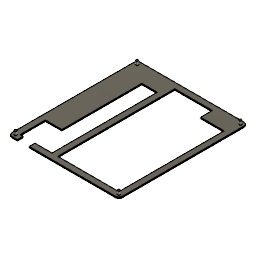
EasySplit-Right-Assembled (Autodesk Fusion 360 archive; units mm, degrees)
design "EasySplit-Right-Top"
part number: 2026-04-16-19-10-06-869
Autodesk Fusion 360 part; units mm, degrees
note: some values were not read from the file. Chosen so that the rebuilt part matches the saved one: a side.
(part 1 of 2)
sketch "Sketch1" plane through (0, 0, 0) normal (0, 0, 1) x (1, 0, 0)
  line L0 (167.6875, -193.6438) -> (-20, -193.6438)
  line L1 (-10, 15) -> (157.6875, 15)
  line L2 (-20, -193.6438) -> (-20, 25)
  line L3 (167.6875, 25) -> (167.6875, -193.6438)
  line L4 (-10, -183.6438) -> (-10, 15)
  line L5 (157.6875, 15) -> (157.6875, -183.6438)
  line L6 (157.6875, -183.6438) -> (-10, -183.6438)
  line L7 (-20, 25) -> (167.6875, 25)
  line L8 (15, -183.6438) -> (-5, -183.6438)
  line L9 (-5, -183.6438) -> (-5, -193.6438)
  line L10 (-5, -193.6438) -> (15, -193.6438)
  line L11 (15, -193.6438) -> (15, -183.6438)
  line L12 (-10, 15) -> (18, 15)
  line L13 (18, 15) -> (18, -141)
  line L14 (18, -141) -> (-10, -141)
  line L15 (-10, -141) -> (-10, 15)
  line L16 (44, 15) -> (54, 15)
  line L17 (54, 15) -> (54, -185)
  line L18 (54, -185) -> (44, -185)
  line L19 (44, -185) -> (44, 15)
  line L20 (157.6875, -183.6438) -> (121.6875, -183.6438)
  line L21 (121.6875, -183.6438) -> (121.6875, -148.1438)
  line L22 (121.6875, -148.1438) -> (157.6875, -148.1438)
  line L23 (157.6875, -148.1438) -> (157.6875, -183.6438)
  line L24 (18, -141) -> (44, -141)
  line L25 (14, -141) -> (18, -141)
  line L26 (18, 15) -> (44, 15)
  line L27 (44, 15) -> (44, -5)
  line L28 (44, -5) -> (18, -5)
  line L29 (18, -5) -> (18, 15)
  line L30 (157.6875, 15) -> (117.6875, 15)
  line L31 (117.6875, 15) -> (117.6875, -5)
  line L32 (117.6875, -5) -> (157.6875, -5)
  line L33 (157.6875, -5) -> (157.6875, 15)
  dimension "d3" = 167.6875
  dimension "d4" = 198.6438
  dimension "d5" = 187.6875
  dimension "d6" = 218.6438
  dimension "d7" = 10
  dimension "d8" = 10
  dimension "d19" = 20
  dimension "d20" = 15
  dimension "d21" = 28
  dimension "d22" = 156
  dimension "d23" = 10
  dimension "d24" = 200
  dimension "d25" = 26
  dimension "d26" = 36
  dimension "d27" = 35.5
  dimension "d29" = 10
  dimension "d30" = 20
  dimension "d31" = 40
  dimension "d32" = 20
  constraint horizontal L1
  constraint vertical L5
  constraint horizontal L6
  constraint vertical L4
  constraint horizontal L7
  constraint vertical L3
  constraint horizontal L0
  constraint vertical L2
  constraint horizontal L8
  constraint vertical L9
  constraint horizontal L10
  constraint vertical L11
  constraint coincident L6 L8.start
  constraint horizontal L12
  constraint vertical L13
  constraint horizontal L14
  constraint vertical L15
  constraint horizontal L16
  constraint vertical L17
  constraint horizontal L18
  constraint vertical L19
  constraint coincident L1 L16.start
  constraint horizontal L20
  constraint vertical L21
  constraint horizontal L22
  constraint vertical L23
  constraint horizontal L24
  constraint horizontal L25
  constraint coincident L14 L25.start
  constraint horizontal L26
  constraint vertical L27
  constraint horizontal L28
  constraint vertical L29
  constraint horizontal L30
  constraint vertical L31
  constraint horizontal L32
  constraint vertical L33
  measures "d3" distance of L1.start L1.end
  measures "d4" distance of L1.start L4.start
  measures "d5" distance of L2.end L3.start
  measures "d6" distance of L2.end L0.end
  measures "d7" distance of L1 L7
  measures "d8" distance of L2 L4
  measures "d19" distance of L8.start L8.end
  measures "d20" distance of L2 L9
  measures "d21" distance of L1.start L12.end
  measures "d22" distance of L1.start L14.end
  measures "d23" distance of L16.start L16.end
  measures "d24" distance of L16.start L18.end
  measures "d25" distance of L13 L19
  measures "d26" distance of L5.end L20.end
  measures "d27" distance of L5.end L22.end
  measures "d29" distance of L8.start L10.end
  measures "d30" distance of L12.end L28.end
  measures "d31" distance of L1.end L30.end
  measures "d32" distance of L1.end L32.end
extrude "Extrude1" add sketch "Sketch1" along normal blind 2 contours L0 L1 L2 L3 L4 L5 L6 L7 L9 L11 L12 L15 L16 L17 L18 L19 L20 L23 L26 L30 L33 | L1 L6 L16 L17 L19 L27 | L6 L17 L18 L19 | L1 L4 L12 L13 L14 L15 L25 L29 | L1 L13 L19 L26 L27 L28 L29 | L1 L5 L30 L31 L32 L33
fillet "Fillet1" radius 6 1 edges at (167.6875, -193.6438, 1)
fillet "Fillet2" radius 6 1 edges at (167.6875, 25, 1)
fillet "Fillet3" radius 6 1 edges at (-20, 25, 1)
fillet "Fillet4" radius 6 1 edges at (-20, -193.6438, 1)
move_face "MoveFace1" to x (-1, 0, 0) y (0, 1, 0) z (0, 0, -1) at (108, 0, 4) 1 faces at (-4, -42.3333, 2)
sketch "Sketch2" plane through (0, 0, 2) normal (0, 0, 1) x (-1, 0, 0)
  arc A0 (20, 187.6438) -> (14, 193.6438) centre (14, 187.6438) ccw
  line L0 (14, 193.6438) -> (5, 193.6438)
  line L1 (5, 193.6438) -> (5, 183.6438)
  line L2 (5, 183.6438) -> (10, 183.6438)
  line L3 (10, 183.6438) -> (10, 141)
  line L4 (10, 141) -> (-18, 141)
  line L5 (-18, 141) -> (-18, 5)
  line L6 (-18, 5) -> (-44, 5)
  line L7 (-44, 5) -> (-44, 183.6438)
  line L8 (-44, 183.6438) -> (-15, 183.6438)
  line L9 (-15, 183.6438) -> (-15, 193.6438)
  line L10 (-15, 193.6438) -> (-161.6875, 193.6438)
  arc A1 (-161.6875, 193.6438) -> (-167.6875, 187.6438) centre (-161.6875, 187.6438) ccw
  line L11 (-167.6875, 187.6438) -> (-167.6875, -19)
  arc A2 (-167.6875, -19) -> (-161.6875, -25) centre (-161.6875, -19) ccw
  line L12 (-161.6875, -25) -> (14, -25)
  arc A3 (14, -25) -> (20, -19) centre (14, -19) ccw
  line L13 (20, -19) -> (20, 187.6438)
  line L14 (-54, 183.6438) -> (-54, -15)
  line L15 (-54, -15) -> (-117.6875, -15)
  line L16 (-117.6875, -15) -> (-117.6875, 5)
  line L17 (-117.6875, 5) -> (-157.6875, 5)
  line L18 (-157.6875, 5) -> (-157.6875, 183.6438)
  line L19 (-157.6875, 183.6438) -> (-54, 183.6438)
  circle A4 centre (14, -19) radius 2.1
  circle A5 centre (-161.6875, -19) radius 2.1
  circle A6 centre (-161.6875, 187.6438) radius 2.1
  circle A7 centre (14, 187.6438) radius 2.1
  dimension "d33" = 4.2
  dimension "d34" = 4.2
  dimension "d35" = 4.2
  dimension "d36" = 4.2
  dimension "d37" = 6
  dimension "d38" = 6
  dimension "d39" = 6
  dimension "d40" = 6
  dimension "d41" = 6
  dimension "d42" = 6
  dimension "d43" = 6
  dimension "d44" = 6
  measures "d33" diameter of A4
  measures "d34" diameter of A5
  measures "d35" diameter of A6
  measures "d36" diameter of A7
  measures "d37" distance of L0 A0.centre
  measures "d38" distance of L13 A0.centre
  measures "d39" distance of L13 A3.centre
  measures "d40" distance of L12 A3.centre
  measures "d41" distance of L11 A2.centre
  measures "d42" distance of L12 A2.centre
  measures "d43" distance of L10 A1.centre
  measures "d44" distance of L11 A1.centre
extrude "Extrude2" add sketch "Sketch2" along normal blind 6 contours A4 | A5 | A6 | A7

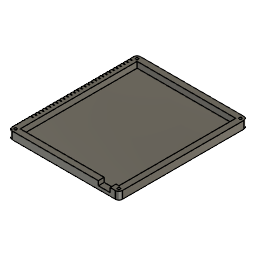
design "EasySplit-Right"
part number: 2026-04-16-18-11-24-138
Autodesk Fusion 360 part; units mm, degrees
sketch "Sketch1" plane through (0, 0, 0) normal (0, 0, 1) x (1, 0, 0)
  line L0 (-10, 15) -> (157.6875, 15)
  line L1 (157.6875, 15) -> (157.6875, -183.6438)
  line L2 (157.6875, -183.6438) -> (-10, -183.6438)
  line L3 (-10, -183.6438) -> (-10, 15)
  line L4 (-20, 25) -> (167.6875, 25)
  line L5 (167.6875, 25) -> (167.6875, -193.6438)
  line L6 (167.6875, -193.6438) -> (-20, -193.6438)
  line L7 (-20, -193.6438) -> (-20, 25)
  dimension "d1" = 167.6875
  dimension "d2" = 198.6438
  dimension "d3" = 187.6875
  dimension "d4" = 218.6438
  dimension "d5" = 10
  dimension "d6" = 10
  constraint horizontal L0
  constraint vertical L1
  constraint horizontal L2
  constraint vertical L3
  constraint horizontal L4
  constraint vertical L5
  constraint horizontal L6
  constraint vertical L7
  measures "d1" distance of L0.start L0.end
  measures "d2" distance of L0.start L2.end
  measures "d3" distance of L4.start L4.end
  measures "d4" distance of L4.start L6.end
  measures "d5" distance of L0 L4
  measures "d6" distance of L3 L7
extrude "Extrude1" add sketch "Sketch1" along normal blind 3 contours L0 L1 L2 L3
extrude "Extrude2" add sketch "Sketch1" along normal blind 13
sketch "Sketch2" plane through (0, 0, 13) normal (0, 0, 1) x (-1, 0, 0)
  line L0 (-157.6875, 183.6438) -> (10, 183.6438)
  line L1 (10, 183.6438) -> (10, -15)
  line L2 (10, -15) -> (-157.6875, -15)
  line L3 (-157.6875, -15) -> (-157.6875, 183.6438)
  line L4 (20, 193.6438) -> (-167.6875, 193.6438)
  line L5 (-167.6875, 193.6438) -> (-167.6875, -25)
  line L6 (-167.6875, -25) -> (20, -25)
  line L7 (20, -25) -> (20, 193.6438)
  line L8 (20, -25) -> (-167.6875, -25)
  line L9 (-132.6875, 183.6438) -> (-152.6875, 183.6438)
  line L10 (-152.6875, 183.6438) -> (-152.6875, 193.6438)
  line L11 (-152.6875, 193.6438) -> (-132.6875, 193.6438)
  line L12 (-132.6875, 193.6438) -> (-132.6875, 183.6438)
  line L13 (20, 193.6438) -> (20, -25)
  dimension "d15" = 20
  dimension "d21" = 15
  constraint horizontal L9
  constraint vertical L10
  constraint horizontal L11
  constraint vertical L12
  constraint coincident L0 L9.start
  measures "d15" distance of L9.start L9.end
  measures "d21" distance of L5 L10
extrude "Extrude4" cut sketch "Sketch2" against normal blind 7.5 contours L0 L4 L9 L10 L11 L12
fillet "Fillet1" radius 6 4 edges at (-20, -193.6438, 6.5) (167.6875, -193.6438, 6.5) (167.6875, 25, 6.5) (-20, 25, 6.5)
sketch "Sketch3" plane through (-20, 0, 0) normal (-1, 0, 0) x (0, -1, 0)
  line L0 (-19, 13) -> (-19, 0)
  line L1 (-19, 0) -> (187.6438, 0)
  line L2 (187.6438, 0) -> (187.6438, 13)
  line L3 (187.6438, 13) -> (-19, 13)
  line L4 (149, 0) -> (156.5042, 12.9976)
  line L5 (23, 0) -> (30.5042, 12.9976)
  line L6 (167, 0) -> (174.5042, 12.9976)
  line L7 (179, 0) -> (186.5042, 12.9976)
  line L8 (77, 0) -> (84.5042, 12.9976)
  line L9 (113, 0) -> (120.5042, 12.9976)
  line L10 (71, 0) -> (78.5042, 12.9976)
  line L11 (41, 0) -> (48.5042, 12.9976)
  line L12 (173, 0) -> (180.5042, 12.9976)
  line L13 (143, 0) -> (150.5042, 12.9976)
  line L14 (65, 0) -> (72.5042, 12.9976)
  line L15 (131, 0) -> (138.5042, 12.9976)
  line L16 (29, 0) -> (36.5042, 12.9976)
  line L17 (101, 0) -> (108.5042, 12.9976)
  line L18 (107, 0) -> (114.5042, 12.9976)
  line L19 (35, 0) -> (42.5042, 12.9976)
  line L20 (47, 0) -> (54.5042, 12.9976)
  line L21 (53, 0) -> (60.5042, 12.9976)
  line L22 (59, 0) -> (66.5042, 12.9976)
  line L23 (137, 0) -> (144.5042, 12.9976)
  line L24 (155, 0) -> (162.5042, 12.9976)
  line L25 (89, 0) -> (96.5042, 12.9976)
  line L26 (161, 0) -> (168.5042, 12.9976)
  line L27 (83, 0) -> (90.5042, 12.9976)
  line L28 (125, 0) -> (132.5042, 12.9976)
  line L29 (95, 0) -> (102.5042, 12.9976)
  line L30 (119, 0) -> (126.5042, 12.9976)
  line L31 (17, 0) -> (24.5042, 12.9976)
  line L32 (11, 0) -> (18.5042, 12.9976)
  line L33 (5, 0) -> (12.5042, 12.9976)
  line L34 (-1, 0) -> (6.5042, 12.9976)
  line L35 (-7, 0) -> (0.5042, 12.9976)
  line L36 (-13, 0) -> (-5.4958, 12.9976)
  line L37 (-19, 0) -> (-11.4958, 12.9976)
  line L38 (185, 0) -> (192.5042, 12.9976)
  spline S0 degree 2 poles (-161.6453, 5.852) (-161.6453, 5.4239) (-161.4102, 5.1797) knots 0 0 0 1 1 1
  spline S1 degree 2 poles (-158.3964, 3.5539) (-158.3964, 3.399) (-158.3281, 3.2729) knots 0 0 0 1 1 1
  spline S2 degree 2 poles (-160.7602, 4.9354) (-160.3925, 4.9354) (-160.1219, 5.156) knots 0 0 0 1 1 1
  spline S3 degree 2 poles (-171.3603, 5.7785) (-171.3603, 6.6006) (-170.8621, 7.2256) knots 0 0 0 1 1 1
  spline S4 degree 2 poles (-158.8179, 7.9781) (-158.9269, 8.0871) (-158.9926, 8.3839) knots 0 0 0 1 1 1
  spline S5 degree 2 poles (-171.1933, 5.118) (-171.3603, 5.3661) (-171.3603, 5.7785) knots 0 0 0 1 1 1
  line L39 (-149.6321, 8.0608) -> (-148.2454, 8.0608)
  spline S6 degree 2 poles (-150.1259, 8.2426) (-150.0051, 8.6482) (-149.837, 8.7997) knots 0 0 0 1 1 1
  line L40 (-150.2782, 7.722) -> (-150.7221, 7.722)
  spline S7 degree 2 poles (-152.3531, 8.4044) (-152.1771, 8.4123) (-151.8475, 8.5819) knots 0 0 0 1 1 1
  line L41 (-152.3898, 8.4071) -> (-152.3531, 8.4044)
  spline S8 degree 2 poles (-156.29, 5.4712) (-156.8022, 4.9354) (-157.5061, 4.9354) knots 0 0 0 1 1 1
  spline S9 degree 2 poles (-158.4095, 8.2552) (-157.9237, 8.2552) (-157.4745, 8.4338) knots 0 0 0 1 1 1
  spline S10 degree 2 poles (-157.5061, 4.9354) (-157.8869, 4.9354) (-158.139, 5.0983) knots 0 0 0 1 1 1
  line L42 (-157.4745, 8.4338) -> (-157.6768, 7.42)
  line L43 (-150.575, 8.0608) -> (-150.1784, 8.0608)
  spline S11 degree 2 poles (-154.575, 6.3773) (-154.6564, 5.9518) (-154.6564, 5.7916) knots 0 0 0 1 1 1
  spline S12 degree 2 poles (-152.8468, 7.3523) (-152.5054, 7.431) (-152.4187, 7.431) knots 0 0 0 1 1 1
  spline S13 degree 2 poles (-164.0195, 7.1258) (-164.5842, 6.3694) (-165.4929, 5.8599) knots 0 0 0 1 1 1
  spline S14 degree 2 poles (-165.1147, 3.9348) (-164.3452, 3.9348) (-163.6439, 4.9512) knots 0 0 0 1 1 1
  spline S15 degree 2 poles (-164.248, 3.8783) (-164.7917, 3.4436) (-165.183, 3.4436) knots 0 0 0 1 1 1
  line L44 (-165.8632, 6.506) -> (-165.6295, 6.0805)
  spline S16 degree 2 poles (-166.6459, 7.1626) (-166.6459, 7.6616) (-166.0655, 7.9663) knots 0 0 0 1 1 1
  spline S17 degree 2 poles (-166.9795, 4.6176) (-167.1659, 4.7542) (-167.1659, 4.9459) knots 0 0 0 1 1 1
  spline S18 degree 2 poles (-165.4036, 5.4791) (-165.4036, 5.0772) (-165.7398, 4.7791) knots 0 0 0 1 1 1
  spline S19 degree 2 poles (-166.7116, 4.9801) (-166.7116, 4.7647) (-166.399, 4.7647) knots 0 0 0 1 1 1
  spline S20 degree 2 poles (-166.9099, 5.3609) (-166.6538, 5.571) (-166.0523, 5.8599) knots 0 0 0 1 1 1
  spline S21 degree 2 poles (-166.399, 4.7647) (-166.1679, 4.7647) (-166.0235, 4.921) knots 0 0 0 1 1 1
  line L45 (-166.0523, 5.8599) -> (-166.2625, 6.1987)
  spline S22 degree 2 poles (-165.9394, 5.6235) (-166.7116, 5.2086) (-166.7116, 4.9801) knots 0 0 0 1 1 1
  line L46 (-166.5277, 7.2309) -> (-166.3229, 7.0891)
  spline S23 degree 2 poles (-165.4929, 5.8599) (-165.4036, 5.6603) (-165.4036, 5.4791) knots 0 0 0 1 1 1
  spline S24 degree 2 poles (-167.1659, 4.9459) (-167.1659, 5.1508) (-166.9099, 5.3609) knots 0 0 0 1 1 1
  spline S25 degree 2 poles (-166.2625, 6.1987) (-166.6459, 6.8159) (-166.6459, 7.1626) knots 0 0 0 1 1 1
  spline S26 degree 2 poles (-165.7398, 4.7791) (-166.076, 4.4811) (-166.5277, 4.4811) knots 0 0 0 1 1 1
  spline S27 degree 2 poles (-166.0655, 7.9663) (-165.7083, 7.8297) (-165.7083, 7.6222) knots 0 0 0 1 1 1
  spline S28 degree 2 poles (-160.8153, 7.9584) (-160.8153, 7.764) (-160.7431, 7.6616) knots 0 0 0 1 1 1
  line L47 (-158.139, 5.0983) -> (-158.3307, 4.1265)
  spline S29 degree 2 poles (-159.8514, 5.6734) (-159.8514, 5.9912) (-160.4476, 6.548) knots 0 0 0 1 1 1
  spline S30 degree 2 poles (-161.2907, 7.764) (-161.2907, 8.2683) (-160.8967, 8.594) knots 0 0 0 1 1 1
  spline S31 degree 2 poles (-160.965, 4.6281) (-161.4141, 4.6281) (-161.707, 4.8382) knots 0 0 0 1 1 1
  line L48 (-160.4476, 6.548) -> (-160.7365, 6.8159)
  spline S32 degree 2 poles (-160.7365, 6.8159) (-161.2907, 7.3307) (-161.2907, 7.764) knots 0 0 0 1 1 1
  spline S33 degree 2 poles (-163.6807, 6.7608) (-163.4049, 6.007) (-163.2684, 5.395) knots 0 0 0 1 1 1
  spline S34 degree 2 poles (-158.9926, 8.3839) (-158.8009, 8.2552) (-158.4095, 8.2552) knots 0 0 0 1 1 1
  line L49 (-164.2296, 7.2545) -> (-164.0195, 7.1258)
  spline S35 degree 2 poles (-159.313, 8.2053) (-159.5415, 8.6465) (-160.0563, 8.6465) knots 0 0 0 1 1 1
  spline S36 degree 2 poles (-158.4804, 7.8691) (-158.7089, 7.8691) (-158.8179, 7.9781) knots 0 0 0 1 1 1
  spline S37 degree 2 poles (-158.097, 7.9164) (-158.3255, 7.8691) (-158.4804, 7.8691) knots 0 0 0 1 1 1
  spline S38 degree 2 poles (-160.1219, 5.156) (-159.8514, 5.3767) (-159.8514, 5.6734) knots 0 0 0 1 1 1
  spline S39 degree 2 poles (-164.2664, 7.5592) (-164.0904, 7.5592) (-163.9736, 7.4003) knots 0 0 0 1 1 1
  spline S40 degree 2 poles (-161.9998, 5.3688) (-161.9998, 5.5868) (-161.6453, 5.852) knots 0 0 0 1 1 1
  spline S41 degree 2 poles (-158.3281, 3.2729) (-158.5934, 3.1862) (-158.7326, 3.1862) knots 0 0 0 1 1 1
  spline S42 degree 2 poles (-161.707, 4.8382) (-161.9998, 5.0484) (-161.9998, 5.3688) knots 0 0 0 1 1 1
  spline S43 degree 2 poles (-158.9506, 3.4331) (-158.9506, 3.6248) (-158.8639, 4.0608) knots 0 0 0 1 1 1
  spline S44 degree 2 poles (-160.8967, 8.594) (-160.5028, 8.9197) (-159.8934, 8.9197) knots 0 0 0 1 1 1
  spline S45 degree 2 poles (-159.8934, 8.9197) (-159.5704, 8.9197) (-159.3708, 8.8212) knots 0 0 0 1 1 1
  spline S46 degree 2 poles (-159.8541, 4.9945) (-160.2953, 4.6281) (-160.965, 4.6281) knots 0 0 0 1 1 1
  spline S47 degree 2 poles (-173.6059, 4.8382) (-174.4647, 4.8382) (-174.4647, 5.4082) knots 0 0 0 1 1 1
  spline S48 degree 2 poles (-167.4338, 5.6432) (-168.0589, 5.0641) (-168.508, 5.0641) knots 0 0 0 1 1 1
  line L50 (-173.5887, 7.2046) -> (-173.0456, 7.2046)
  line L51 (-173.3275, 8.4994) -> (-173.5887, 7.2046)
  spline S49 degree 2 poles (-167.4955, 6.0241) (-167.0031, 6.4981) (-166.5277, 7.2309) knots 0 0 0 1 1 1
  line L52 (-172.4803, 8.4994) -> (-173.3275, 8.4994)
  spline S50 degree 2 poles (-173.1935, 5.2585) (-172.5212, 5.2585) (-172.009, 5.4975) knots 0 0 0 1 1 1
  spline S51 degree 2 poles (-172.9755, 4.8973) (-173.3852, 4.8382) (-173.6059, 4.8382) knots 0 0 0 1 1 1
  line L53 (-174.2257, 7.2046) -> (-174.139, 7.2046)
  spline S52 degree 2 poles (-173.8711, 5.6078) (-173.8711, 5.2585) (-173.1935, 5.2585) knots 0 0 0 1 1 1
  spline S53 degree 2 poles (-172.4003, 5.0116) (-172.5658, 4.9564) (-172.9755, 4.8973) knots 0 0 0 1 1 1
  spline S54 degree 2 poles (-174.4988, 8.7306) (-174.3202, 8.8225) (-173.3984, 8.8225) knots 0 0 0 1 1 1
  line L54 (-173.8816, 8.4994) -> (-173.9578, 8.4994)
  line L55 (-174.2047, 6.879) -> (-174.2441, 6.879)
  spline S55 degree 2 poles (-174.5212, 7.1258) (-174.4279, 7.2046) (-174.2257, 7.2046) knots 0 0 0 1 1 1
  spline S56 degree 2 poles (-174.4647, 5.4082) (-174.4647, 5.5605) (-174.3806, 5.9939) knots 0 0 0 1 1 1
  spline S57 degree 2 poles (-170.4826, 5.3714) (-170.1065, 5.3714) (-169.044, 7.0208) knots 0 0 0 1 1 1
  spline S58 degree 2 poles (-170.5404, 7.0457) (-170.8298, 6.5638) (-170.8298, 5.9019) knots 0 0 0 1 1 1
  spline S59 degree 2 poles (-159.4128, 5.9177) (-159.4128, 5.3609) (-159.8541, 4.9945) knots 0 0 0 1 1 1
  spline S60 degree 2 poles (-160.7431, 7.6616) (-160.6709, 7.5592) (-160.2953, 7.2151) knots 0 0 0 1 1 1
  spline S61 degree 2 poles (-163.9736, 7.4003) (-163.8567, 7.2414) (-163.6807, 6.7608) knots 0 0 0 1 1 1
  spline S62 degree 2 poles (-161.4102, 5.1797) (-161.1751, 4.9354) (-160.7602, 4.9354) knots 0 0 0 1 1 1
  spline S63 degree 2 poles (-164.0445, 6.3445) (-164.3321, 7.0339) (-164.6656, 7.3964) knots 0 0 0 1 1 1
  spline S64 degree 2 poles (-160.596, 8.4482) (-160.8153, 8.2499) (-160.8153, 7.9584) knots 0 0 0 1 1 1
  spline S65 degree 2 poles (-161.8475, 7.5434) (-161.8475, 7.2913) (-162.2611, 6.506) knots 0 0 0 1 1 1
  spline S66 degree 2 poles (-159.3708, 8.8212) (-159.1712, 8.7227) (-159.1712, 8.5651) knots 0 0 0 1 1 1
  spline S67 degree 2 poles (-163.6439, 4.9512) (-163.7569, 5.6551) (-164.0445, 6.3445) knots 0 0 0 1 1 1
  spline S68 degree 2 poles (-164.8731, 6.594) (-164.6183, 6.808) (-164.2296, 7.2545) knots 0 0 0 1 1 1
  spline S69 degree 2 poles (-162.2611, 6.506) (-162.6748, 5.7207) (-163.1528, 5.0667) knots 0 0 0 1 1 1
  line L56 (-158.8639, 4.0608) -> (-158.097, 7.9164)
  spline S70 degree 2 poles (-169.7092, 7.8507) (-169.3122, 7.8507) (-168.8495, 7.6038) knots 0 0 0 1 1 1
  spline S71 degree 2 poles (-170.8621, 7.2256) (-170.3639, 7.8507) (-169.7092, 7.8507) knots 0 0 0 1 1 1
  spline S72 degree 2 poles (-170.8298, 5.9019) (-170.8298, 5.3714) (-170.4826, 5.3714) knots 0 0 0 1 1 1
  spline S73 degree 2 poles (-168.1902, 7.8455) (-168.3399, 7.617) (-168.4187, 7.2204) knots 0 0 0 1 1 1
  spline S74 degree 2 poles (-169.044, 7.0208) (-169.0308, 7.0418) (-168.9361, 7.1679) knots 0 0 0 1 1 1
  spline S75 degree 2 poles (-169.8891, 5.357) (-170.3822, 4.8698) (-170.7476, 4.8698) knots 0 0 0 1 1 1
  spline S76 degree 2 poles (-170.7476, 4.8698) (-171.0264, 4.8698) (-171.1933, 5.118) knots 0 0 0 1 1 1
  spline S77 degree 2 poles (-168.2927, 7.8481) (-168.2611, 7.8481) (-168.1902, 7.8455) knots 0 0 0 1 1 1
  spline S78 degree 2 poles (-168.9361, 7.1679) (-169.4885, 7.5277) (-169.854, 7.5277) knots 0 0 0 1 1 1
  spline S79 degree 2 poles (-168.8495, 7.6038) (-168.7812, 7.8481) (-168.2927, 7.8481) knots 0 0 0 1 1 1
  line L57 (-168.4187, 7.2204) -> (-168.4634, 6.9971)
  spline S80 degree 2 poles (-169.0753, 6.0096) (-169.0753, 6.2066) (-169.0596, 6.5401) knots 0 0 0 1 1 1
  spline S81 degree 2 poles (-168.2716, 5.55) (-167.988, 5.55) (-167.4955, 6.0241) knots 0 0 0 1 1 1
  spline S82 degree 2 poles (-168.508, 5.0641) (-169.0753, 5.0641) (-169.0753, 6.0096) knots 0 0 0 1 1 1
  spline S83 degree 2 poles (-168.4634, 6.9971) (-168.5395, 6.6242) (-168.5395, 6.1252) knots 0 0 0 1 1 1
  spline S84 degree 2 poles (-169.854, 7.5277) (-170.2511, 7.5277) (-170.5404, 7.0457) knots 0 0 0 1 1 1
  spline S85 degree 2 poles (-168.5395, 6.1252) (-168.5395, 5.55) (-168.2716, 5.55) knots 0 0 0 1 1 1
  spline S86 degree 2 poles (-169.0596, 6.5401) (-169.3961, 5.8442) (-169.8891, 5.357) knots 0 0 0 1 1 1
  spline S87 degree 2 poles (-165.6295, 6.0805) (-165.1279, 6.3799) (-164.8731, 6.594) knots 0 0 0 1 1 1
  line L58 (-173.6521, 6.879) -> (-173.7867, 6.204)
  spline S88 degree 2 poles (-147.6886, 8.1557) (-147.7542, 7.8866) (-147.8632, 7.8043) knots 0 0 0 1 1 1
  spline S89 degree 2 poles (-172.6157, 8.8225) (-171.8751, 8.8225) (-171.4128, 8.9696) knots 0 0 0 1 1 1
  spline S90 degree 2 poles (-152.4187, 7.431) (-152.2244, 7.431) (-152.2244, 7.1581) knots 0 0 0 1 1 1
  spline S91 degree 2 poles (-172.4553, 6.9472) (-172.5944, 6.879) (-173.1088, 6.879) knots 0 0 0 1 1 1
  line L59 (-174.139, 7.2046) -> (-173.8816, 8.4994)
  spline S92 degree 2 poles (-173.0456, 7.2046) (-172.4762, 7.2046) (-172.1377, 7.3491) knots 0 0 0 1 1 1
  spline S93 degree 2 poles (-173.7867, 6.204) (-173.8711, 5.7837) (-173.8711, 5.6078) knots 0 0 0 1 1 1
  spline S94 degree 2 poles (-152.2244, 7.1581) (-152.2244, 6.9561) (-152.3005, 6.5782) knots 0 0 0 1 1 1
  spline S95 degree 2 poles (-150.0523, 7.0847) (-150.6459, 6.0442) (-151.2526, 5.457) knots 0 0 0 1 1 1
  spline S96 degree 2 poles (-151.3314, 8.9275) (-151.447, 8.5651) (-151.7411, 8.3208) knots 0 0 0 1 1 1
  line L60 (-173.3984, 8.8225) -> (-172.6157, 8.8225)
  line L61 (-150.2703, 7.2132) -> (-150.0523, 7.0847)
  spline S97 degree 2 poles (-151.1659, 7.6432) (-151.0136, 7.9199) (-150.9138, 7.9904) knots 0 0 0 1 1 1
  spline S98 degree 2 poles (-173.9578, 8.4994) (-174.4437, 8.4994) (-174.8586, 8.1895) knots 0 0 0 1 1 1
  spline S99 degree 2 poles (-152.3452, 7.9479) (-152.4502, 7.9479) (-152.4502, 8.0765) knots 0 0 0 1 1 1
  line L62 (-173.1088, 6.879) -> (-173.6521, 6.879)
  spline S100 degree 2 poles (-152.4502, 8.0765) (-152.4502, 8.2601) (-152.3898, 8.4071) knots 0 0 0 1 1 1
  spline S101 degree 2 poles (-149.2066, 8.9459) (-149.4115, 8.6825) (-149.6321, 8.0608) knots 0 0 0 1 1 1
  line L63 (-150.1784, 8.0608) -> (-150.1259, 8.2426)
  spline S102 degree 2 poles (-148.2454, 8.0608) (-147.8803, 8.0608) (-147.6886, 8.1557) knots 0 0 0 1 1 1
  spline S103 degree 2 poles (-151.8475, 8.5819) (-151.5179, 8.7514) (-151.3314, 8.9275) knots 0 0 0 1 1 1
  spline S104 degree 2 poles (-149.7451, 7.722) (-149.7713, 7.6354) (-149.7845, 7.5933) knots 0 0 0 1 1 1
  spline S105 degree 2 poles (-149.837, 8.7997) (-149.6689, 8.9512) (-149.3327, 8.9512) knots 0 0 0 1 1 1
  spline S106 degree 2 poles (-171.4128, 8.9696) (-171.62, 8.6413) (-171.7813, 8.5704) knots 0 0 0 1 1 1
  line L64 (-152.6498, 7.2204) -> (-152.4397, 7.0759)
  spline S107 degree 2 poles (-174.2441, 6.879) (-174.5093, 6.879) (-174.7588, 6.7634) knots 0 0 0 1 1 1
  spline S108 degree 2 poles (-150.9138, 7.9904) (-150.814, 8.0608) (-150.575, 8.0608) knots 0 0 0 1 1 1
  spline S109 degree 2 poles (-171.7813, 8.5704) (-171.9426, 8.4994) (-172.4803, 8.4994) knots 0 0 0 1 1 1
  line L65 (-148.269, 7.722) -> (-149.7451, 7.722)
  spline S110 degree 2 poles (-172.1377, 7.3491) (-172.3162, 7.0155) (-172.4553, 6.9472) knots 0 0 0 1 1 1
  spline S111 degree 2 poles (-152.4397, 7.0759) (-152.9834, 6.0438) (-153.5323, 5.4568) knots 0 0 0 1 1 1
  spline S112 degree 2 poles (-174.8586, 8.1895) (-174.7273, 8.6097) (-174.4988, 8.7306) knots 0 0 0 1 1 1
  spline S113 degree 2 poles (-172.009, 5.4975) (-172.1272, 5.1035) (-172.4003, 5.0116) knots 0 0 0 1 1 1
  spline S114 degree 2 poles (-150.659, 5.8757) (-150.659, 6.3694) (-150.399, 7.2808) knots 0 0 0 1 1 1
  line L66 (-174.3806, 5.9939) -> (-174.2047, 6.879)
  spline S115 degree 2 poles (-152.8862, 6.2306) (-152.7575, 6.8558) (-152.7575, 7.108) knots 0 0 0 1 1 1
  spline S116 degree 2 poles (-151.3288, 5.8134) (-150.7825, 6.3657) (-150.2703, 7.2132) knots 0 0 0 1 1 1
  spline S117 degree 2 poles (-174.7588, 6.7634) (-174.6144, 7.047) (-174.5212, 7.1258) knots 0 0 0 1 1 1
  spline S118 degree 2 poles (-149.7845, 7.5933) (-150.1022, 6.5113) (-150.1022, 5.9597) knots 0 0 0 1 1 1
  spline S119 degree 2 poles (-150.7221, 7.722) (-151.0005, 7.722) (-151.1659, 7.6432) knots 0 0 0 1 1 1
  spline S120 degree 2 poles (-151.7411, 8.3208) (-152.1876, 7.9479) (-152.3452, 7.9479) knots 0 0 0 1 1 1
  line L67 (-157.7556, 7.0155) -> (-158.0576, 5.5053)
  spline S121 degree 2 poles (-147.8632, 7.8043) (-147.9722, 7.722) (-148.269, 7.722) knots 0 0 0 1 1 1
  spline S122 degree 2 poles (-156.7523, 7.8507) (-156.3347, 7.8507) (-156.0563, 7.5342) knots 0 0 0 1 1 1
  line L68 (-155.3708, 9.4581) -> (-155.3708, 9.5185)
  spline S123 degree 2 poles (-156.0563, 7.5342) (-155.7779, 7.2178) (-155.7779, 6.745) knots 0 0 0 1 1 1
  spline S124 degree 2 poles (-155.7779, 6.745) (-155.7779, 6.007) (-156.29, 5.4712) knots 0 0 0 1 1 1
  spline S125 degree 2 poles (-154.3307, 5.3478) (-154.0156, 5.3478) (-153.6965, 5.7036) knots 0 0 0 1 1 1
  spline S126 degree 2 poles (-154.7667, 8.9538) (-155.3708, 8.9538) (-155.3708, 9.4581) knots 0 0 0 1 1 1
  spline S127 degree 2 poles (-155.3708, 9.5185) (-155.0556, 9.3399) (-154.659, 9.3399) knots 0 0 0 1 1 1
  spline S128 degree 2 poles (-149.3327, 8.9512) (-149.2933, 8.9512) (-149.2066, 8.9459) knots 0 0 0 1 1 1
  line L69 (-150.399, 7.2808) -> (-150.2782, 7.722)
  spline S129 degree 2 poles (-152.7575, 7.108) (-152.7575, 7.2577) (-152.8468, 7.3523) knots 0 0 0 1 1 1
  spline S130 degree 2 poles (-155.1896, 5.7286) (-155.1896, 5.944) (-155.1108, 6.3379) knots 0 0 0 1 1 1
  spline S131 degree 2 poles (-156.6196, 5.5841) (-156.2953, 5.9728) (-156.2953, 6.5296) knots 0 0 0 1 1 1
  spline S132 degree 2 poles (-157.6768, 7.42) (-157.2303, 7.8507) (-156.7523, 7.8507) knots 0 0 0 1 1 1
  spline S133 degree 2 poles (-156.4791, 7.181) (-156.663, 7.4305) (-156.9571, 7.4305) knots 0 0 0 1 1 1
  spline S134 degree 2 poles (-166.0235, 4.921) (-165.879, 5.0772) (-165.879, 5.3241) knots 0 0 0 1 1 1
  spline S135 degree 2 poles (-165.7083, 7.6222) (-165.7083, 7.3281) (-166.1627, 7.0575) knots 0 0 0 1 1 1
  spline S136 degree 2 poles (-166.3229, 7.0891) (-166.8087, 6.2224) (-167.4338, 5.6432) knots 0 0 0 1 1 1
  spline S137 degree 2 poles (-165.183, 3.4436) (-165.5349, 3.4436) (-165.5349, 3.7404) knots 0 0 0 1 1 1
  line L70 (-166.1627, 7.0575) -> (-165.8632, 6.506)
  spline S138 degree 2 poles (-165.4719, 4.0241) (-165.3275, 3.9348) (-165.1147, 3.9348) knots 0 0 0 1 1 1
  spline S139 degree 2 poles (-165.879, 5.3241) (-165.879, 5.4712) (-165.9394, 5.6235) knots 0 0 0 1 1 1
  spline S140 degree 2 poles (-166.5277, 4.4811) (-166.793, 4.4811) (-166.9795, 4.6176) knots 0 0 0 1 1 1
  spline S141 degree 2 poles (-165.5349, 3.7404) (-165.5349, 3.8612) (-165.4719, 4.0241) knots 0 0 0 1 1 1
  spline S142 degree 2 poles (-149.9473, 4.8698) (-150.2625, 4.8698) (-150.4607, 5.1508) knots 0 0 0 1 1 1
  spline S143 degree 2 poles (-151.2526, 5.457) (-151.8593, 4.8698) (-152.3426, 4.8698) knots 0 0 0 1 1 1
  spline S144 degree 2 poles (-152.8166, 5.0615) (-152.9965, 5.2533) (-152.9965, 5.5659) knots 0 0 0 1 1 1
  spline S145 degree 2 poles (-148.7208, 5.7496) (-148.7208, 5.4922) (-149.1554, 5.181) knots 0 0 0 1 1 1
  spline S146 degree 2 poles (-152.3426, 4.8698) (-152.6367, 4.8698) (-152.8166, 5.0615) knots 0 0 0 1 1 1
  spline S147 degree 2 poles (-149.6636, 5.3504) (-149.4378, 5.3504) (-149.1712, 5.5421) knots 0 0 0 1 1 1
  spline S148 degree 2 poles (-159.1712, 8.5651) (-159.1712, 8.4101) (-159.313, 8.2053) knots 0 0 0 1 1 1
  spline S149 degree 2 poles (-149.1712, 5.5421) (-148.9046, 5.7338) (-148.7917, 5.9755) knots 0 0 0 1 1 1
  line L71 (-152.3005, 6.5782) -> (-152.403, 6.0666)
  spline S150 degree 2 poles (-149.1554, 5.181) (-149.5901, 4.8698) (-149.9473, 4.8698) knots 0 0 0 1 1 1
  spline S151 degree 2 poles (-150.1022, 5.9597) (-150.1022, 5.3504) (-149.6636, 5.3504) knots 0 0 0 1 1 1
  spline S152 degree 2 poles (-148.7917, 5.9755) (-148.7208, 5.8468) (-148.7208, 5.7496) knots 0 0 0 1 1 1
  spline S153 degree 2 poles (-152.9965, 5.5659) (-152.9965, 5.6841) (-152.944, 5.9416) knots 0 0 0 1 1 1
  spline S154 degree 2 poles (-152.2034, 5.2611) (-151.8751, 5.2611) (-151.3288, 5.8134) knots 0 0 0 1 1 1
  spline S155 degree 2 poles (-160.0589, 6.9971) (-159.4128, 6.3957) (-159.4128, 5.9177) knots 0 0 0 1 1 1
  spline S156 degree 2 poles (-153.6965, 5.7036) (-153.3774, 6.0595) (-152.6498, 7.2204) knots 0 0 0 1 1 1
  spline S157 degree 2 poles (-164.6656, 7.3964) (-164.4713, 7.5592) (-164.2664, 7.5592) knots 0 0 0 1 1 1
  spline S158 degree 2 poles (-153.5323, 5.4568) (-154.0812, 4.8698) (-154.5041, 4.8698) knots 0 0 0 1 1 1
  spline S159 degree 2 poles (-158.3307, 4.1265) (-158.3964, 3.7982) (-158.3964, 3.5539) knots 0 0 0 1 1 1
  spline S160 degree 2 poles (-160.0563, 8.6465) (-160.3767, 8.6465) (-160.596, 8.4482) knots 0 0 0 1 1 1
  spline S161 degree 2 poles (-163.2684, 5.395) (-162.3806, 6.8002) (-162.3071, 7.8507) knots 0 0 0 1 1 1
  line L72 (-160.2953, 7.2151) -> (-160.0589, 6.9971)
  spline S162 degree 2 poles (-162.3071, 7.8507) (-161.8475, 7.7824) (-161.8475, 7.5434) knots 0 0 0 1 1 1
  spline S163 degree 2 poles (-158.7326, 3.1862) (-158.9506, 3.1862) (-158.9506, 3.4331) knots 0 0 0 1 1 1
  spline S164 degree 2 poles (-163.1528, 5.0667) (-163.7043, 4.313) (-164.248, 3.8783) knots 0 0 0 1 1 1
  line L73 (-152.944, 5.9416) -> (-152.8862, 6.2306)
  spline S165 degree 2 poles (-154.659, 9.3399) (-154.2625, 9.3399) (-153.9657, 9.5369) knots 0 0 0 1 1 1
  spline S166 degree 2 poles (-152.403, 6.0666) (-152.4791, 5.6967) (-152.4791, 5.5864) knots 0 0 0 1 1 1
  spline S167 degree 2 poles (-154.6564, 5.7916) (-154.6564, 5.3478) (-154.3307, 5.3478) knots 0 0 0 1 1 1
  spline S168 degree 2 poles (-158.0576, 5.5053) (-157.7923, 5.1954) (-157.4063, 5.1954) knots 0 0 0 1 1 1
  spline S169 degree 2 poles (-157.4063, 5.1954) (-156.944, 5.1954) (-156.6196, 5.5841) knots 0 0 0 1 1 1
  spline S170 degree 2 poles (-156.9571, 7.4305) (-157.3248, 7.4305) (-157.7556, 7.0155) knots 0 0 0 1 1 1
  spline S171 degree 2 poles (-154.5041, 4.8698) (-154.8114, 4.8698) (-155.0005, 5.1074) knots 0 0 0 1 1 1
  spline S172 degree 2 poles (-152.4791, 5.5864) (-152.4791, 5.2611) (-152.2034, 5.2611) knots 0 0 0 1 1 1
  line L74 (-153.9657, 9.5369) -> (-154.575, 6.3773)
  spline S173 degree 2 poles (-156.2953, 6.5296) (-156.2953, 6.9315) (-156.4791, 7.181) knots 0 0 0 1 1 1
  spline S174 degree 2 poles (-154.5881, 8.9696) (-154.6906, 8.9538) (-154.7667, 8.9538) knots 0 0 0 1 1 1
  spline S175 degree 2 poles (-150.4607, 5.1508) (-150.659, 5.4318) (-150.659, 5.8757) knots 0 0 0 1 1 1
  line L75 (-155.1108, 6.3379) -> (-154.5881, 8.9696)
  spline S176 degree 2 poles (-155.0005, 5.1074) (-155.1896, 5.3451) (-155.1896, 5.7286) knots 0 0 0 1 1 1
  spline S177 degree 2 poles (-161.6453, 5.852) (-161.6453, 5.4239) (-161.4102, 5.1797) knots 0 0 0 1 1 1
  spline S178 degree 2 poles (-158.3964, 3.5539) (-158.3964, 3.399) (-158.3281, 3.2729) knots 0 0 0 1 1 1
  spline S179 degree 2 poles (-160.7602, 4.9354) (-160.3925, 4.9354) (-160.1219, 5.156) knots 0 0 0 1 1 1
  spline S180 degree 2 poles (-171.3603, 5.7785) (-171.3603, 6.6006) (-170.8621, 7.2256) knots 0 0 0 1 1 1
  spline S181 degree 2 poles (-158.8179, 7.9781) (-158.9269, 8.0871) (-158.9926, 8.3839) knots 0 0 0 1 1 1
  spline S182 degree 2 poles (-171.1933, 5.118) (-171.3603, 5.3661) (-171.3603, 5.7785) knots 0 0 0 1 1 1
  line L76 (-149.6321, 8.0608) -> (-148.2454, 8.0608)
  spline S183 degree 2 poles (-150.1259, 8.2426) (-150.0051, 8.6482) (-149.837, 8.7997) knots 0 0 0 1 1 1
  line L77 (-150.2782, 7.722) -> (-150.7221, 7.722)
  spline S184 degree 2 poles (-152.3531, 8.4044) (-152.1771, 8.4123) (-151.8475, 8.5819) knots 0 0 0 1 1 1
  line L78 (-152.3898, 8.4071) -> (-152.3531, 8.4044)
  spline S185 degree 2 poles (-156.29, 5.4712) (-156.8022, 4.9354) (-157.5061, 4.9354) knots 0 0 0 1 1 1
  spline S186 degree 2 poles (-158.4095, 8.2552) (-157.9237, 8.2552) (-157.4745, 8.4338) knots 0 0 0 1 1 1
  spline S187 degree 2 poles (-157.5061, 4.9354) (-157.8869, 4.9354) (-158.139, 5.0983) knots 0 0 0 1 1 1
  line L79 (-157.4745, 8.4338) -> (-157.6768, 7.42)
  line L80 (-150.575, 8.0608) -> (-150.1784, 8.0608)
  spline S188 degree 2 poles (-154.575, 6.3773) (-154.6564, 5.9518) (-154.6564, 5.7916) knots 0 0 0 1 1 1
  spline S189 degree 2 poles (-152.8468, 7.3523) (-152.5054, 7.431) (-152.4187, 7.431) knots 0 0 0 1 1 1
  spline S190 degree 2 poles (-164.0195, 7.1258) (-164.5842, 6.3694) (-165.4929, 5.8599) knots 0 0 0 1 1 1
  spline S191 degree 2 poles (-165.1147, 3.9348) (-164.3452, 3.9348) (-163.6439, 4.9512) knots 0 0 0 1 1 1
  spline S192 degree 2 poles (-164.248, 3.8783) (-164.7917, 3.4436) (-165.183, 3.4436) knots 0 0 0 1 1 1
  line L81 (-165.8632, 6.506) -> (-165.6295, 6.0805)
  spline S193 degree 2 poles (-166.6459, 7.1626) (-166.6459, 7.6616) (-166.0655, 7.9663) knots 0 0 0 1 1 1
  spline S194 degree 2 poles (-166.9795, 4.6176) (-167.1659, 4.7542) (-167.1659, 4.9459) knots 0 0 0 1 1 1
  spline S195 degree 2 poles (-165.4036, 5.4791) (-165.4036, 5.0772) (-165.7398, 4.7791) knots 0 0 0 1 1 1
  spline S196 degree 2 poles (-166.7116, 4.9801) (-166.7116, 4.7647) (-166.399, 4.7647) knots 0 0 0 1 1 1
  spline S197 degree 2 poles (-166.9099, 5.3609) (-166.6538, 5.571) (-166.0523, 5.8599) knots 0 0 0 1 1 1
  spline S198 degree 2 poles (-166.399, 4.7647) (-166.1679, 4.7647) (-166.0235, 4.921) knots 0 0 0 1 1 1
  line L82 (-166.0523, 5.8599) -> (-166.2625, 6.1987)
  spline S199 degree 2 poles (-165.9394, 5.6235) (-166.7116, 5.2086) (-166.7116, 4.9801) knots 0 0 0 1 1 1
  line L83 (-166.5277, 7.2309) -> (-166.3229, 7.0891)
  spline S200 degree 2 poles (-165.4929, 5.8599) (-165.4036, 5.6603) (-165.4036, 5.4791) knots 0 0 0 1 1 1
  spline S201 degree 2 poles (-167.1659, 4.9459) (-167.1659, 5.1508) (-166.9099, 5.3609) knots 0 0 0 1 1 1
  spline S202 degree 2 poles (-166.2625, 6.1987) (-166.6459, 6.8159) (-166.6459, 7.1626) knots 0 0 0 1 1 1
  spline S203 degree 2 poles (-165.7398, 4.7791) (-166.076, 4.4811) (-166.5277, 4.4811) knots 0 0 0 1 1 1
  spline S204 degree 2 poles (-166.0655, 7.9663) (-165.7083, 7.8297) (-165.7083, 7.6222) knots 0 0 0 1 1 1
  spline S205 degree 2 poles (-160.8153, 7.9584) (-160.8153, 7.764) (-160.7431, 7.6616) knots 0 0 0 1 1 1
  line L84 (-158.139, 5.0983) -> (-158.3307, 4.1265)
  spline S206 degree 2 poles (-159.8514, 5.6734) (-159.8514, 5.9912) (-160.4476, 6.548) knots 0 0 0 1 1 1
  spline S207 degree 2 poles (-161.2907, 7.764) (-161.2907, 8.2683) (-160.8967, 8.594) knots 0 0 0 1 1 1
  spline S208 degree 2 poles (-160.965, 4.6281) (-161.4141, 4.6281) (-161.707, 4.8382) knots 0 0 0 1 1 1
  line L85 (-160.4476, 6.548) -> (-160.7365, 6.8159)
  spline S209 degree 2 poles (-160.7365, 6.8159) (-161.2907, 7.3307) (-161.2907, 7.764) knots 0 0 0 1 1 1
  spline S210 degree 2 poles (-163.6807, 6.7608) (-163.4049, 6.007) (-163.2684, 5.395) knots 0 0 0 1 1 1
  spline S211 degree 2 poles (-158.9926, 8.3839) (-158.8009, 8.2552) (-158.4095, 8.2552) knots 0 0 0 1 1 1
  line L86 (-164.2296, 7.2545) -> (-164.0195, 7.1258)
  spline S212 degree 2 poles (-159.313, 8.2053) (-159.5415, 8.6465) (-160.0563, 8.6465) knots 0 0 0 1 1 1
  spline S213 degree 2 poles (-158.4804, 7.8691) (-158.7089, 7.8691) (-158.8179, 7.9781) knots 0 0 0 1 1 1
  spline S214 degree 2 poles (-158.097, 7.9164) (-158.3255, 7.8691) (-158.4804, 7.8691) knots 0 0 0 1 1 1
  spline S215 degree 2 poles (-160.1219, 5.156) (-159.8514, 5.3767) (-159.8514, 5.6734) knots 0 0 0 1 1 1
  spline S216 degree 2 poles (-164.2664, 7.5592) (-164.0904, 7.5592) (-163.9736, 7.4003) knots 0 0 0 1 1 1
  spline S217 degree 2 poles (-161.9998, 5.3688) (-161.9998, 5.5868) (-161.6453, 5.852) knots 0 0 0 1 1 1
  spline S218 degree 2 poles (-158.3281, 3.2729) (-158.5934, 3.1862) (-158.7326, 3.1862) knots 0 0 0 1 1 1
  spline S219 degree 2 poles (-161.707, 4.8382) (-161.9998, 5.0484) (-161.9998, 5.3688) knots 0 0 0 1 1 1
  spline S220 degree 2 poles (-158.9506, 3.4331) (-158.9506, 3.6248) (-158.8639, 4.0608) knots 0 0 0 1 1 1
  spline S221 degree 2 poles (-160.8967, 8.594) (-160.5028, 8.9197) (-159.8934, 8.9197) knots 0 0 0 1 1 1
  spline S222 degree 2 poles (-159.8934, 8.9197) (-159.5704, 8.9197) (-159.3708, 8.8212) knots 0 0 0 1 1 1
  spline S223 degree 2 poles (-159.8541, 4.9945) (-160.2953, 4.6281) (-160.965, 4.6281) knots 0 0 0 1 1 1
  spline S224 degree 2 poles (-173.6059, 4.8382) (-174.4647, 4.8382) (-174.4647, 5.4082) knots 0 0 0 1 1 1
  spline S225 degree 2 poles (-167.4338, 5.6432) (-168.0589, 5.0641) (-168.508, 5.0641) knots 0 0 0 1 1 1
  line L87 (-173.5887, 7.2046) -> (-173.0456, 7.2046)
  line L88 (-173.3275, 8.4994) -> (-173.5887, 7.2046)
  spline S226 degree 2 poles (-167.4955, 6.0241) (-167.0031, 6.4981) (-166.5277, 7.2309) knots 0 0 0 1 1 1
  line L89 (-172.4803, 8.4994) -> (-173.3275, 8.4994)
  spline S227 degree 2 poles (-173.1935, 5.2585) (-172.5212, 5.2585) (-172.009, 5.4975) knots 0 0 0 1 1 1
  spline S228 degree 2 poles (-172.9755, 4.8973) (-173.3852, 4.8382) (-173.6059, 4.8382) knots 0 0 0 1 1 1
  line L90 (-174.2257, 7.2046) -> (-174.139, 7.2046)
  spline S229 degree 2 poles (-173.8711, 5.6078) (-173.8711, 5.2585) (-173.1935, 5.2585) knots 0 0 0 1 1 1
  spline S230 degree 2 poles (-172.4003, 5.0116) (-172.5658, 4.9564) (-172.9755, 4.8973) knots 0 0 0 1 1 1
  spline S231 degree 2 poles (-174.4988, 8.7306) (-174.3202, 8.8225) (-173.3984, 8.8225) knots 0 0 0 1 1 1
  line L91 (-173.8816, 8.4994) -> (-173.9578, 8.4994)
  line L92 (-174.2047, 6.879) -> (-174.2441, 6.879)
  spline S232 degree 2 poles (-174.5212, 7.1258) (-174.4279, 7.2046) (-174.2257, 7.2046) knots 0 0 0 1 1 1
  spline S233 degree 2 poles (-174.4647, 5.4082) (-174.4647, 5.5605) (-174.3806, 5.9939) knots 0 0 0 1 1 1
  spline S234 degree 2 poles (-170.4826, 5.3714) (-170.1065, 5.3714) (-169.044, 7.0208) knots 0 0 0 1 1 1
  spline S235 degree 2 poles (-170.5404, 7.0457) (-170.8298, 6.5638) (-170.8298, 5.9019) knots 0 0 0 1 1 1
  spline S236 degree 2 poles (-159.4128, 5.9177) (-159.4128, 5.3609) (-159.8541, 4.9945) knots 0 0 0 1 1 1
  spline S237 degree 2 poles (-160.7431, 7.6616) (-160.6709, 7.5592) (-160.2953, 7.2151) knots 0 0 0 1 1 1
  spline S238 degree 2 poles (-163.9736, 7.4003) (-163.8567, 7.2414) (-163.6807, 6.7608) knots 0 0 0 1 1 1
  spline S239 degree 2 poles (-161.4102, 5.1797) (-161.1751, 4.9354) (-160.7602, 4.9354) knots 0 0 0 1 1 1
  spline S240 degree 2 poles (-164.0445, 6.3445) (-164.3321, 7.0339) (-164.6656, 7.3964) knots 0 0 0 1 1 1
  spline S241 degree 2 poles (-160.596, 8.4482) (-160.8153, 8.2499) (-160.8153, 7.9584) knots 0 0 0 1 1 1
  spline S242 degree 2 poles (-161.8475, 7.5434) (-161.8475, 7.2913) (-162.2611, 6.506) knots 0 0 0 1 1 1
  spline S243 degree 2 poles (-159.3708, 8.8212) (-159.1712, 8.7227) (-159.1712, 8.5651) knots 0 0 0 1 1 1
  spline S244 degree 2 poles (-163.6439, 4.9512) (-163.7569, 5.6551) (-164.0445, 6.3445) knots 0 0 0 1 1 1
  spline S245 degree 2 poles (-164.8731, 6.594) (-164.6183, 6.808) (-164.2296, 7.2545) knots 0 0 0 1 1 1
  spline S246 degree 2 poles (-162.2611, 6.506) (-162.6748, 5.7207) (-163.1528, 5.0667) knots 0 0 0 1 1 1
  line L93 (-158.8639, 4.0608) -> (-158.097, 7.9164)
  spline S247 degree 2 poles (-169.7092, 7.8507) (-169.3122, 7.8507) (-168.8495, 7.6038) knots 0 0 0 1 1 1
  spline S248 degree 2 poles (-170.8621, 7.2256) (-170.3639, 7.8507) (-169.7092, 7.8507) knots 0 0 0 1 1 1
  spline S249 degree 2 poles (-170.8298, 5.9019) (-170.8298, 5.3714) (-170.4826, 5.3714) knots 0 0 0 1 1 1
  spline S250 degree 2 poles (-168.1902, 7.8455) (-168.3399, 7.617) (-168.4187, 7.2204) knots 0 0 0 1 1 1
  spline S251 degree 2 poles (-169.044, 7.0208) (-169.0308, 7.0418) (-168.9361, 7.1679) knots 0 0 0 1 1 1
  spline S252 degree 2 poles (-169.8891, 5.357) (-170.3822, 4.8698) (-170.7476, 4.8698) knots 0 0 0 1 1 1
  spline S253 degree 2 poles (-170.7476, 4.8698) (-171.0264, 4.8698) (-171.1933, 5.118) knots 0 0 0 1 1 1
  spline S254 degree 2 poles (-168.2927, 7.8481) (-168.2611, 7.8481) (-168.1902, 7.8455) knots 0 0 0 1 1 1
  spline S255 degree 2 poles (-168.9361, 7.1679) (-169.4885, 7.5277) (-169.854, 7.5277) knots 0 0 0 1 1 1
  spline S256 degree 2 poles (-168.8495, 7.6038) (-168.7812, 7.8481) (-168.2927, 7.8481) knots 0 0 0 1 1 1
  line L94 (-168.4187, 7.2204) -> (-168.4634, 6.9971)
  spline S257 degree 2 poles (-169.0753, 6.0096) (-169.0753, 6.2066) (-169.0596, 6.5401) knots 0 0 0 1 1 1
  spline S258 degree 2 poles (-168.2716, 5.55) (-167.988, 5.55) (-167.4955, 6.0241) knots 0 0 0 1 1 1
  spline S259 degree 2 poles (-168.508, 5.0641) (-169.0753, 5.0641) (-169.0753, 6.0096) knots 0 0 0 1 1 1
  spline S260 degree 2 poles (-168.4634, 6.9971) (-168.5395, 6.6242) (-168.5395, 6.1252) knots 0 0 0 1 1 1
  spline S261 degree 2 poles (-169.854, 7.5277) (-170.2511, 7.5277) (-170.5404, 7.0457) knots 0 0 0 1 1 1
  spline S262 degree 2 poles (-168.5395, 6.1252) (-168.5395, 5.55) (-168.2716, 5.55) knots 0 0 0 1 1 1
  spline S263 degree 2 poles (-169.0596, 6.5401) (-169.3961, 5.8442) (-169.8891, 5.357) knots 0 0 0 1 1 1
  spline S264 degree 2 poles (-165.6295, 6.0805) (-165.1279, 6.3799) (-164.8731, 6.594) knots 0 0 0 1 1 1
  line L95 (-173.6521, 6.879) -> (-173.7867, 6.204)
  spline S265 degree 2 poles (-147.6886, 8.1557) (-147.7542, 7.8866) (-147.8632, 7.8043) knots 0 0 0 1 1 1
  spline S266 degree 2 poles (-172.6157, 8.8225) (-171.8751, 8.8225) (-171.4128, 8.9696) knots 0 0 0 1 1 1
  spline S267 degree 2 poles (-152.4187, 7.431) (-152.2244, 7.431) (-152.2244, 7.1581) knots 0 0 0 1 1 1
  spline S268 degree 2 poles (-172.4553, 6.9472) (-172.5944, 6.879) (-173.1088, 6.879) knots 0 0 0 1 1 1
  line L96 (-174.139, 7.2046) -> (-173.8816, 8.4994)
  spline S269 degree 2 poles (-173.0456, 7.2046) (-172.4762, 7.2046) (-172.1377, 7.3491) knots 0 0 0 1 1 1
  spline S270 degree 2 poles (-173.7867, 6.204) (-173.8711, 5.7837) (-173.8711, 5.6078) knots 0 0 0 1 1 1
  spline S271 degree 2 poles (-152.2244, 7.1581) (-152.2244, 6.9561) (-152.3005, 6.5782) knots 0 0 0 1 1 1
  spline S272 degree 2 poles (-150.0523, 7.0847) (-150.6459, 6.0442) (-151.2526, 5.457) knots 0 0 0 1 1 1
  spline S273 degree 2 poles (-151.3314, 8.9275) (-151.447, 8.5651) (-151.7411, 8.3208) knots 0 0 0 1 1 1
  line L97 (-173.3984, 8.8225) -> (-172.6157, 8.8225)
  line L98 (-150.2703, 7.2132) -> (-150.0523, 7.0847)
  spline S274 degree 2 poles (-151.1659, 7.6432) (-151.0136, 7.9199) (-150.9138, 7.9904) knots 0 0 0 1 1 1
  spline S275 degree 2 poles (-173.9578, 8.4994) (-174.4437, 8.4994) (-174.8586, 8.1895) knots 0 0 0 1 1 1
  spline S276 degree 2 poles (-152.3452, 7.9479) (-152.4502, 7.9479) (-152.4502, 8.0765) knots 0 0 0 1 1 1
  line L99 (-173.1088, 6.879) -> (-173.6521, 6.879)
  spline S277 degree 2 poles (-152.4502, 8.0765) (-152.4502, 8.2601) (-152.3898, 8.4071) knots 0 0 0 1 1 1
  spline S278 degree 2 poles (-149.2066, 8.9459) (-149.4115, 8.6825) (-149.6321, 8.0608) knots 0 0 0 1 1 1
  line L100 (-150.1784, 8.0608) -> (-150.1259, 8.2426)
  spline S279 degree 2 poles (-148.2454, 8.0608) (-147.8803, 8.0608) (-147.6886, 8.1557) knots 0 0 0 1 1 1
  spline S280 degree 2 poles (-151.8475, 8.5819) (-151.5179, 8.7514) (-151.3314, 8.9275) knots 0 0 0 1 1 1
  spline S281 degree 2 poles (-149.7451, 7.722) (-149.7713, 7.6354) (-149.7845, 7.5933) knots 0 0 0 1 1 1
  spline S282 degree 2 poles (-149.837, 8.7997) (-149.6689, 8.9512) (-149.3327, 8.9512) knots 0 0 0 1 1 1
  spline S283 degree 2 poles (-171.4128, 8.9696) (-171.62, 8.6413) (-171.7813, 8.5704) knots 0 0 0 1 1 1
  line L101 (-152.6498, 7.2204) -> (-152.4397, 7.0759)
  spline S284 degree 2 poles (-174.2441, 6.879) (-174.5093, 6.879) (-174.7588, 6.7634) knots 0 0 0 1 1 1
  spline S285 degree 2 poles (-150.9138, 7.9904) (-150.814, 8.0608) (-150.575, 8.0608) knots 0 0 0 1 1 1
  spline S286 degree 2 poles (-171.7813, 8.5704) (-171.9426, 8.4994) (-172.4803, 8.4994) knots 0 0 0 1 1 1
  line L102 (-148.269, 7.722) -> (-149.7451, 7.722)
  spline S287 degree 2 poles (-172.1377, 7.3491) (-172.3162, 7.0155) (-172.4553, 6.9472) knots 0 0 0 1 1 1
  spline S288 degree 2 poles (-152.4397, 7.0759) (-152.9834, 6.0438) (-153.5323, 5.4568) knots 0 0 0 1 1 1
  spline S289 degree 2 poles (-174.8586, 8.1895) (-174.7273, 8.6097) (-174.4988, 8.7306) knots 0 0 0 1 1 1
  spline S290 degree 2 poles (-172.009, 5.4975) (-172.1272, 5.1035) (-172.4003, 5.0116) knots 0 0 0 1 1 1
  spline S291 degree 2 poles (-150.659, 5.8757) (-150.659, 6.3694) (-150.399, 7.2808) knots 0 0 0 1 1 1
  line L103 (-174.3806, 5.9939) -> (-174.2047, 6.879)
  spline S292 degree 2 poles (-152.8862, 6.2306) (-152.7575, 6.8558) (-152.7575, 7.108) knots 0 0 0 1 1 1
  spline S293 degree 2 poles (-151.3288, 5.8134) (-150.7825, 6.3657) (-150.2703, 7.2132) knots 0 0 0 1 1 1
  spline S294 degree 2 poles (-174.7588, 6.7634) (-174.6144, 7.047) (-174.5212, 7.1258) knots 0 0 0 1 1 1
  spline S295 degree 2 poles (-149.7845, 7.5933) (-150.1022, 6.5113) (-150.1022, 5.9597) knots 0 0 0 1 1 1
  spline S296 degree 2 poles (-150.7221, 7.722) (-151.0005, 7.722) (-151.1659, 7.6432) knots 0 0 0 1 1 1
  spline S297 degree 2 poles (-151.7411, 8.3208) (-152.1876, 7.9479) (-152.3452, 7.9479) knots 0 0 0 1 1 1
  line L104 (-157.7556, 7.0155) -> (-158.0576, 5.5053)
  spline S298 degree 2 poles (-147.8632, 7.8043) (-147.9722, 7.722) (-148.269, 7.722) knots 0 0 0 1 1 1
  spline S299 degree 2 poles (-156.7523, 7.8507) (-156.3347, 7.8507) (-156.0563, 7.5342) knots 0 0 0 1 1 1
  line L105 (-155.3708, 9.4581) -> (-155.3708, 9.5185)
  spline S300 degree 2 poles (-156.0563, 7.5342) (-155.7779, 7.2178) (-155.7779, 6.745) knots 0 0 0 1 1 1
  spline S301 degree 2 poles (-155.7779, 6.745) (-155.7779, 6.007) (-156.29, 5.4712) knots 0 0 0 1 1 1
  spline S302 degree 2 poles (-154.3307, 5.3478) (-154.0156, 5.3478) (-153.6965, 5.7036) knots 0 0 0 1 1 1
  spline S303 degree 2 poles (-154.7667, 8.9538) (-155.3708, 8.9538) (-155.3708, 9.4581) knots 0 0 0 1 1 1
  spline S304 degree 2 poles (-155.3708, 9.5185) (-155.0556, 9.3399) (-154.659, 9.3399) knots 0 0 0 1 1 1
  spline S305 degree 2 poles (-149.3327, 8.9512) (-149.2933, 8.9512) (-149.2066, 8.9459) knots 0 0 0 1 1 1
  line L106 (-150.399, 7.2808) -> (-150.2782, 7.722)
  spline S306 degree 2 poles (-152.7575, 7.108) (-152.7575, 7.2577) (-152.8468, 7.3523) knots 0 0 0 1 1 1
  spline S307 degree 2 poles (-155.1896, 5.7286) (-155.1896, 5.944) (-155.1108, 6.3379) knots 0 0 0 1 1 1
  spline S308 degree 2 poles (-156.6196, 5.5841) (-156.2953, 5.9728) (-156.2953, 6.5296) knots 0 0 0 1 1 1
  spline S309 degree 2 poles (-157.6768, 7.42) (-157.2303, 7.8507) (-156.7523, 7.8507) knots 0 0 0 1 1 1
  spline S310 degree 2 poles (-156.4791, 7.181) (-156.663, 7.4305) (-156.9571, 7.4305) knots 0 0 0 1 1 1
  spline S311 degree 2 poles (-166.0235, 4.921) (-165.879, 5.0772) (-165.879, 5.3241) knots 0 0 0 1 1 1
  spline S312 degree 2 poles (-165.7083, 7.6222) (-165.7083, 7.3281) (-166.1627, 7.0575) knots 0 0 0 1 1 1
  spline S313 degree 2 poles (-166.3229, 7.0891) (-166.8087, 6.2224) (-167.4338, 5.6432) knots 0 0 0 1 1 1
  spline S314 degree 2 poles (-165.183, 3.4436) (-165.5349, 3.4436) (-165.5349, 3.7404) knots 0 0 0 1 1 1
  line L107 (-166.1627, 7.0575) -> (-165.8632, 6.506)
  spline S315 degree 2 poles (-165.4719, 4.0241) (-165.3275, 3.9348) (-165.1147, 3.9348) knots 0 0 0 1 1 1
  spline S316 degree 2 poles (-165.879, 5.3241) (-165.879, 5.4712) (-165.9394, 5.6235) knots 0 0 0 1 1 1
  spline S317 degree 2 poles (-166.5277, 4.4811) (-166.793, 4.4811) (-166.9795, 4.6176) knots 0 0 0 1 1 1
  spline S318 degree 2 poles (-165.5349, 3.7404) (-165.5349, 3.8612) (-165.4719, 4.0241) knots 0 0 0 1 1 1
  spline S319 degree 2 poles (-149.9473, 4.8698) (-150.2625, 4.8698) (-150.4607, 5.1508) knots 0 0 0 1 1 1
  spline S320 degree 2 poles (-151.2526, 5.457) (-151.8593, 4.8698) (-152.3426, 4.8698) knots 0 0 0 1 1 1
  spline S321 degree 2 poles (-152.8166, 5.0615) (-152.9965, 5.2533) (-152.9965, 5.5659) knots 0 0 0 1 1 1
  spline S322 degree 2 poles (-148.7208, 5.7496) (-148.7208, 5.4922) (-149.1554, 5.181) knots 0 0 0 1 1 1
  spline S323 degree 2 poles (-152.3426, 4.8698) (-152.6367, 4.8698) (-152.8166, 5.0615) knots 0 0 0 1 1 1
  spline S324 degree 2 poles (-149.6636, 5.3504) (-149.4378, 5.3504) (-149.1712, 5.5421) knots 0 0 0 1 1 1
  spline S325 degree 2 poles (-159.1712, 8.5651) (-159.1712, 8.4101) (-159.313, 8.2053) knots 0 0 0 1 1 1
  spline S326 degree 2 poles (-149.1712, 5.5421) (-148.9046, 5.7338) (-148.7917, 5.9755) knots 0 0 0 1 1 1
  line L108 (-152.3005, 6.5782) -> (-152.403, 6.0666)
  spline S327 degree 2 poles (-149.1554, 5.181) (-149.5901, 4.8698) (-149.9473, 4.8698) knots 0 0 0 1 1 1
  spline S328 degree 2 poles (-150.1022, 5.9597) (-150.1022, 5.3504) (-149.6636, 5.3504) knots 0 0 0 1 1 1